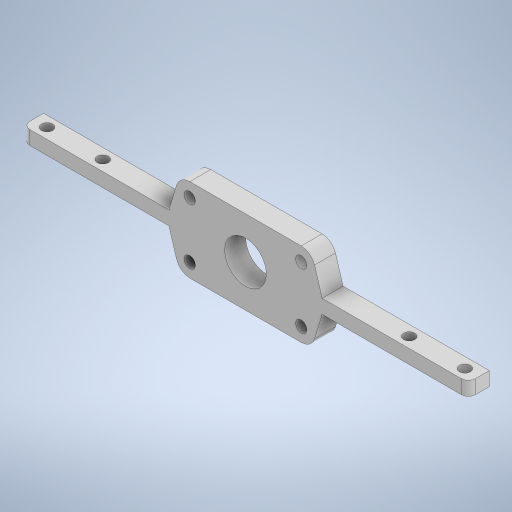
# Autodesk Inventor part: Face Plate
Saved by Autodesk Inventor 2023 (Build 270158000, 158)
## iProperties
Created: 2023-02-27
Part Number: Face Plate
Material: Generic
Document SubType Name: Modeling
Designer: Gabriel - T3 CAD
Density: 1 g/cm^3
Appearance: Default
Author: Gabriel - T3 CAD
Autodesk Inventor part; units mm, degrees
ref_plane "YZ Plane" through (0, 0, 0) normal (1, 0, 0) x (0, 1, 0)
ref_plane "XZ Plane" through (0, 0, 0) normal (0, 1, 0) x (-1, 0, 0)
ref_plane "XY Plane" through (0, 0, 0) normal (0, 0, 1) x (1, 0, 0)
sketch "Sketch1" plane through (0, 0, 0) normal (0, 1, 0) x (-1, 0, 0)
  line L0 (0, 0) -> (203.2, 0)
  line L1 (203.2, 0) -> (203.2, 6.35)
  line L2 (34.925, 9.525) -> (3.175, 9.525)
  line L3 (0, 6.35) -> (0, 0)
  circle A0 centre (6.35, 4.7625) radius 2.5797
  circle A1 centre (31.75, 4.7625) radius 2.5797
  circle A2 centre (171.45, 4.7625) radius 2.5797
  circle A3 centre (196.85, 4.7625) radius 2.5797
  line L4 (38.1, 9.525) -> (165.1, 9.525)
  line L5 (165.1, 6.35) -> (165.1, 4.7625)
  line L6 (38.1, 4.7625) -> (38.1, 6.35)
  arc A4 (38.1, 6.35) -> (34.925, 9.525) centre (34.925, 6.35) ccw
  arc A5 (3.175, 9.525) -> (0, 6.35) centre (3.175, 6.35) ccw
  line L7 (168.275, 9.525) -> (200.025, 9.525)
  arc A6 (168.275, 9.525) -> (165.1, 6.35) centre (168.275, 6.35) ccw
  arc A7 (203.2, 6.35) -> (200.025, 9.525) centre (200.025, 6.35) ccw
  line L8 (165.1, 6.35) -> (165.1, 0)
  line L9 (38.1, 6.35) -> (38.1, 0)
  line L10 (165.1, 4.7625) -> (165.1, 9.525)
  line L11 (168.275, 9.525) -> (165.1, 9.525)
  line L12 (38.1, 6.35) -> (38.1, 9.525)
  line L13 (38.1, 9.525) -> (34.925, 9.525)
  line L14 (38.1, 3.175) -> (165.1, 3.175)
  line L15 (139.7, 3.175) -> (167.578, 9.4476)
  line L16 (63.5, 3.175) -> (35.622, 9.4476)
  point P0 (203.2, 9.525)
  point P1 (0, 9.525)
  dimension "d0" = 203.2
  dimension "d1" = 9.525
  dimension "d2" = 4.7625
  dimension "d3" = 4.7625
  dimension "d4" = 4.7625
  dimension "d5" = 4.7625
  dimension "d6" = 25.4
  dimension "d7" = 25.4
  dimension "d8" = 5.1594
  dimension "d9" = 6.35
  dimension "d10" = 6.35
  dimension "d11" = 4.7625
  dimension "d12" = 6.35
  dimension "d13" = 6.35
  dimension "d14" = 3.175
  dimension "d15" = 3.175
  dimension "d37" = 3.175
  dimension "d100" = 25.4
  constraints: 34 end point, 13 point on line, 12 tangent, 10 point on circle, 8 centre point, 7 perpendicular, 5 equal radius, 3 horizontal, 3 midpoint, 3 parallel, 1 equal length
  measures "d0" distance of point (203.2, 9.525) point (0, 9.525)
  measures "d1" distance of L0.end point (203.2, 9.525)
  measures "d2" distance from line of L0 A0.centre
  measures "d3" distance from line of L0 A1.centre
  measures "d4" distance from line of L0 A2.centre
  measures "d5" distance from line of L0 A3.centre
  measures "d6" distance of A0.centre A1.centre
  measures "d7" distance of A2.centre A3.centre
  measures "d8" diameter of A3
  measures "d9" distance from line of L3 A0.centre
  measures "d10" distance from line of L1 A3.centre
  measures "d11" distance of L6.start L4.start
  measures "d12" distance from line of A1.centre L6
  measures "d13" distance from line of A2.centre L5
  measures "d14" radius of A4
  measures "d15" radius of A6
  measures "d37" distance between parallel lines of L14 L0
  measures "d100" distance of point (165.1, 3.175) L15.start
extrude "Extrusion1" add sketch "Sketch1" along normal mid plane 6.35
extrude "Extrusion2" add sketch "Sketch1" along normal mid plane 50.8 contours L9 L14 L8 L0 | L9 L6 L12 L16 L14 | L14 L15 L10 L5 L8 | L16 L12 L4 L10 L15 L14
sketch "Sketch4" plane through (-38.1, 25.4, 0) normal (0, 0, -1) x (-1, 0, 0)
  line L0 (101.6, -50.8) -> (101.6, -28.575)
  line L1 (25.4, 0) -> (101.6, 0)
  line L2 (101.6, 0) -> (101.6, -50.8)
  line L3 (101.6, -50.8) -> (25.4, -50.8)
  line L4 (25.4, -50.8) -> (25.4, 0)
  circle A0 centre (63.5, -25.4) radius 9.525
  circle A1 centre (38.1, -12.7) radius 2.5797
  circle A2 centre (38.1, -38.1) radius 2.5797
  circle A3 centre (88.9, -12.7) radius 2.5797
  circle A4 centre (88.9, -38.1) radius 2.5797
  circle A5 centre (38.1, -12.7) radius 6.35
  circle A6 centre (38.1, -38.1) radius 6.35
  circle A7 centre (88.9, -12.7) radius 6.35
  circle A8 centre (88.9, -38.1) radius 6.35
  line L5 (38.1, -6.35) -> (88.9, -6.35)
  line L6 (95.25, -11.1925) -> (95.25, -39.6075)
  line L7 (88.9, -44.45) -> (38.1, -44.45)
  line L8 (31.75, -39.6075) -> (31.75, -11.1925)
  line L9 (-38.1, -22.225) -> (31.75, -22.225)
  line L10 (31.75, -22.225) -> (31.75, -28.575)
  line L11 (31.75, -28.575) -> (-38.1, -28.575)
  line L12 (-38.1, -28.575) -> (-38.1, -22.225)
  line L13 (95.25, -22.225) -> (165.1, -22.225)
  line L14 (165.1, -22.225) -> (165.1, -28.575)
  line L15 (165.1, -28.575) -> (95.25, -28.575)
  line L16 (95.25, -28.575) -> (95.25, -22.225)
  line L17 (-38.1, -28.575) -> (-38.1, -22.225) projected
  line L18 (165.1, -28.575) -> (-38.1, -28.575) projected
  line L19 (28.575, -22.225) -> (32.0234, -10.8567)
  line L20 (28.575, -28.575) -> (32.0234, -39.9433)
  line L21 (94.9766, -10.8567) -> (98.425, -22.225)
  line L22 (98.425, -28.575) -> (94.9766, -39.9433)
  line L23 (0, -22.225) -> (0, 0) projected
  line L24 (0, 0) -> (127, 0)
  line L25 (127, 0) -> (127, -50.8)
  line L26 (127, -50.8) -> (0, -50.8)
  line L27 (0, -50.8) -> (0, 0)
  point P0 (-38.1, -25.4)
  point P1 (76.2, -28.575)
  point P2 (-38.1, -25.4)
  point P3 (32.4276, -9.8458)
  point P4 (0, -28.575)
  point P5 (32.4276, -40.9542)
  point P6 (94.5724, -9.8458)
  point P7 (94.5724, -40.9542)
  point P8 (76.2, -28.575)
  point P9 (76.2, -28.575)
  point P10 (25.4, -28.575)
  point P11 (25.4, -22.225)
  point P12 (101.6, -28.575)
  point P13 (-38.1, -50.8)
  point P14 (-38.1, 0)
  point P15 (101.6, -28.575)
  point P16 (101.6, -28.575)
  point P17 (0, -28.575)
  point P18 (25.4, -50.8)
  point P19 (25.4, 0)
  point P20 (127, -22.225)
  point P21 (127, -28.575)
  dimension "d71" = 76.2
  dimension "d72" = 50.8
  dimension "d73" = 25.4
  dimension "d74" = 38.1
  dimension "d75" = 19.05
  dimension "d78" = 25.4
  dimension "d81" = 50.8
  dimension "d84" = 12.7
  dimension "d85" = 12.7
  dimension "d86" = 5.1594
  dimension "d87" = 12.7
  dimension "d90" = 25.4
  dimension "d93" = 50.8
  dimension "d96" = 3.175
  dimension "d97" = 6.35
  dimension "d111" = 3.175
  dimension "d112" = 63.5
  dimension "d113" = 15.875
  dimension "d114" = 0
  dimension "d115" = 17.3825
  dimension "d116" = 11.0325
  dimension "d117" = 94.5724
  dimension "d118" = 94.5724
  dimension "d119" = 76.2
  dimension "d120" = 0
  dimension "d121" = 32.4276
  dimension "d122" = 32.4276
  dimension "d123" = 17.3825
  dimension "d124" = 11.0325
  constraints: 46 end point, 12 point on circle, 9 centre point, 9 parallel, 8 tangent, 7 horizontal, 6 point on line, 5 perpendicular, 4 collinear, 4 equal length, 2 coincident, 2 equal radius, 2 midpoint, 2 vertical alignment, 1 vertical, 14 other
  measures "d72" distance between parallel lines of L1 L3
  measures "d73" distance from line of L3 point (63.5, -25.4)
  measures "d75" diameter of A0
  measures "d78" distance of A1.centre A2.centre
  measures "d81" distance of A1.centre A3.centre
  measures "d84" distance from line of L1 A1.centre
  measures "d86" diameter of A1
  measures "d87" diameter of A5
  measures "d90" distance of A5.centre A6.centre
  measures "d93" distance of A5.centre A7.centre
  measures "d96" distance from line of A0.centre L11
  measures "d97" distance of L11.end L9.start
  measures "d111" distance of L9.end L19.start
  measures "d112" distance from line of L23 A0.centre
  measures "d113" distance between parallel lines of L7 L18
  measures "d114" distance from line of point (101.6, -28.575) L18
  measures "d115" distance from line of L6.start L18
  measures "d116" distance from line of L6.end L18
  measures "d117" distance from line of A7.start L23
  measures "d118" distance from line of A8.start L23
  measures "d119" distance from line of point (76.2, -28.575) L23
  measures "d120" distance from line of point (76.2, -28.575) L18
  measures "d121" distance from line of A5.start L23
  measures "d122" distance from line of A6.start L23
  measures "d123" distance from line of L8.end L18
  measures "d124" distance from line of L8.start L18
extrude "Extrusion5" cut sketch "Sketch4" against normal through all contours L3 L4 L11 L20 A6 L7 A8 L22 L15 L0 | L0 L15 L25 L26 | L26 L27 L11 L4 | L13 L21 A7 L5 A5 L19 L9 L4 L1 L2 | L2 L24 L25 L13 | L9 L23 L24 L4 | L18 A0 | A0 L18 | A1 | A2 | A3 | A4
equation "\"d2\" = 0.5 * d1"
equation "\"d3\" = d2"
equation "\"d4\" = d2"
equation "\"d5\" = d2"
equation "\"d10\" = d9"
equation "\"d11\" = 0.5 * d1"
equation "\"d37\" = 0.333333 * d1"
body "Solid1"
